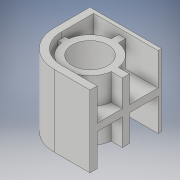
# Autodesk Inventor part: straight_beam_inner_part
Saved by Autodesk Inventor 2019.3 (Build 233278000, 278)
## iProperties
Created: 2019-01-31
Part Number: straight_beam_inner_part
Material: Generic
Document SubType Name: Modeling
Designer: Varga Daniel
Density: 1 g/cm^3
Appearance: Default
Author: Varga Daniel
Autodesk Inventor part; units mm, degrees
ref_plane "YZ Plane" through (0, 0, 0) normal (1, 0, 0) x (0, 1, 0)
ref_plane "XZ Plane" through (0, 0, 0) normal (0, 1, 0) x (-1, 0, 0)
ref_plane "XY Plane" through (0, 0, 0) normal (0, 0, 1) x (1, 0, 0)
derived "Base_part.ipt"
sketch "Beam_sketch" plane through (0, 0, 0) normal (0, 1, 0) x (-1, 0, 0)
  line L0 (5, 0) -> (25, 0)
  line L1 (30, 5) -> (30, 25)
  line L2 (25, 30) -> (5, 30)
  line L3 (0, 25) -> (0, 5)
  line L4 (5, 29) -> (25, 29)
  line L5 (29, 25) -> (29, 5)
  line L6 (25, 1) -> (5, 1)
  line L7 (1, 5) -> (1, 25)
  circle A0 centre (5, 5) radius 2.5
  circle A1 centre (5, 5) radius 3.5
  arc A2 (25, 0) -> (30, 5) centre (25, 5) ccw
  arc A3 (30, 25) -> (25, 30) centre (25, 25) ccw
  arc A4 (5, 30) -> (0, 25) centre (5, 25) ccw
  arc A5 (0, 5) -> (5, 0) centre (5, 5) ccw
  arc A6 (1, 5) -> (5, 1) centre (5, 5) ccw
  arc A7 (5, 29) -> (1, 25) centre (5, 25) ccw
  arc A8 (29, 25) -> (25, 29) centre (25, 25) ccw
  arc A9 (25, 1) -> (29, 5) centre (25, 5) ccw
  line L8 (49.1041, 15) -> (-27.081, 15) construction
  line L9 (31.1478, 10) -> (-2.4877, 10) construction
  line L10 (-2.8604, 5) -> (35.495, 5) construction
  line L11 (5, -2.5736) -> (5, 36.7522) construction
  line L12 (15, -1.4978) -> (15, 34.8784) construction
  line L13 (1.5359, 5.5) -> (1, 5.5)
  line L14 (1.5359, 4.5) -> (1.0314, 4.5)
  line L15 (28.9686, 4.5) -> (8.4641, 4.5)
  line L16 (29, 5.5) -> (8.4641, 5.5)
  line L17 (4.5, 1.5359) -> (4.5, 1.0314)
  line L18 (5.5, 1.5359) -> (5.5, 1)
  line L19 (29, 10.5) -> (1, 10.5)
  line L20 (29, 9.5) -> (1, 9.5)
  line L21 (4.5, 28.9686) -> (4.5, 10.5)
  line L22 (4.5, 9.5) -> (4.5, 8.4641)
  line L23 (5.5, 29) -> (5.5, 10.5)
  line L24 (5.5, 9.5) -> (5.5, 8.4641)
  point P0 (0, 0)
  point P1 (30, 30)
  point P2 (0, 30)
sketch "Sketch3" plane through (0, 0, 0) normal (0, 1, 0) x (-1, 0, 0)
  circle A0 centre (5, 5) radius 2.5 construction
  circle A1 centre (5, 5) radius 3.5 construction
  circle A2 centre (5, 5) radius 2.5
  circle A3 centre (5, 5) radius 3.5
  line L0 (0.3508, 5) -> (13.598, 5) construction
  line L1 (5, 13.9543) -> (5, -1.7484) construction
  line L2 (5, 10) -> (0, 10)
  line L3 (0, 10) -> (0, 9)
  line L4 (0, 9) -> (4.5, 9)
  line L5 (9, 0.5) -> (0, 0.5)
  line L6 (0, 0.5) -> (0, 0)
  line L7 (0, 0) -> (10, 0)
  line L8 (0, 0) -> (0, 9)
  line L9 (1.5359, 5.5) -> (0, 5.5)
  line L10 (0, 5.5) -> (0, 4.5)
  line L11 (0, 4.5) -> (1.5359, 4.5)
  line L12 (5.5, 8.9686) -> (5.5, 8.4641)
  line L13 (4.5, 9) -> (4.5, 8.4641)
  line L14 (4.5, 1.5359) -> (4.5, 0.5)
  line L15 (4.5, 9) -> (5, 9)
  line L16 (0, 9) -> (0, 10)
  line L17 (9, 4.5) -> (8.4641, 4.5)
  arc A4 (10, 5) -> (5, 10) centre (5, 5) ccw
  arc A5 (9, 5) -> (5, 9) centre (5, 5) ccw
  line L18 (8.4641, 5.5) -> (8.9686, 5.5)
  line L19 (5.5, 1.5359) -> (5.5, 0.5)
  line L20 (5, 0) -> (10, 0)
  line L21 (10, 0) -> (10, 5)
  line L22 (9, 5) -> (9, 0.5)
  point P0 (0, 0)
  point P1 (5, 0.5)
  dimension "d4" = 0.5
  dimension "d5" = 1
  dimension "d7" = 1
  dimension "d20" = 5
  dimension "d21" = 5
  dimension "d22" = 1
  dimension "d26" = 5
  dimension "d41" = 10
  dimension "d42" = 4
  constraints: 46 end point, 15 point on line, 8 perpendicular, 6 point on circle, 4 collinear, 4 horizontal, 4 parallel, 3 centre point, 3 midpoint, 2 coincident, 2 tangent, 2 vertical, 1 concentric, 13 other
  measures "d4" distance between parallel lines of L5 L7
  measures "d5" distance between parallel lines of L2 L4
  measures "d7" distance between parallel lines of L12 L13
  measures "d20" distance between parallel lines of L0 L7
  measures "d21" distance between parallel lines of L2 L0
  measures "d22" distance between parallel lines of L9 L11
  measures "d26" radius of A4
  measures "d41" distance between parallel lines of L8 L21
  measures "d42" radius of A5
ref_plane "Work Plane2" through (-5, 0, 0) normal (0, 1, 0) x (-1, 0, 0)
extrude "Extrusion7" add sketch "Sketch3" along normal blind 5 contours A5 L15 L4 L3 L2 A4 L21 L7 L6 L5 L22
extrude "Extrusion8" add sketch "Sketch3" against normal blind 5 contours A5 L15 L4 L3 L2 A4 L21 L7 L6 L5 L22
extrude "Extrusion9" add sketch "Sketch3" along normal blind 4.2 contours A3 | A3 L18 A5 L22 L17 | A3 L13 L15 A5 L12 | L19 L5 L14 A3 | A3 L11 L8 L9
extrude "Extrusion10" add sketch "Sketch3" against normal blind 4.2 contours A3 | A3 L18 A5 L22 L17 | A3 L13 L15 A5 L12 | L19 L5 L14 A3 | A3 L11 L8 L9
extrude "Extrusion11" add sketch "Sketch3" along normal blind 0.5 contours A3 L12 A5 L18 | L17 L22 L5 L19 A3 | A5 L15 L4 L3 L2 A4 L21 L7 L6 L5 L22 | A3 L9 L8 L4 L13 | L14 L5 L8 L11 A3
extrude "Extrusion12" add sketch "Sketch3" against normal blind 0.5 contours A3 L12 A5 L18 | L17 L22 L5 L19 A3 | A5 L15 L4 L3 L2 A4 L21 L7 L6 L5 L22 | A3 L9 L8 L4 L13 | L14 L5 L8 L11 A3
ref_plane "Work Plane3" through (-5, 5, 10) normal (1, 0, 0) x (0, 0, -1)
equation "\"d4\" = 0.5 * Wall_thickness"
equation "\"d5\" = Width_tolerance + Wall_thickness"
equation "\"d7\" = Inner_route_thickness"
equation "\"d22\" = Inner_route_thickness"
equation "\"d28\" = 0.5 * Overall_height"
equation "\"d30\" = 0.5 * Overall_height"
equation "\"d32\" = 0.5 * Hole_height"
equation "\"d34\" = 0.5 * Hole_height"
equation "\"d36\" = 0.5 * Inner_thickness"
equation "\"d38\" = 0.5 * Inner_thickness"
equation "\"d6\" = Inner_route_thickness"
equation "\"Wall_thickness\" = 1"
equation "\"Width_tolerance\" = 0"
equation "\"Inner_route_thickness\" = 1"
equation "\"Overall_height\" = 10"
equation "\"Hole_height\" = 8.4"
equation "\"Inner_thickness\" = 1"
body "Solid2"
